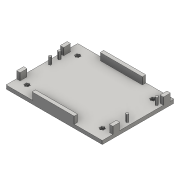
# Autodesk Inventor part: ROB-L-J-1
Saved by Autodesk Inventor 2016 (Build 200138000, 138)
## iProperties
Created: 2016-02-16
Part Number: ROB-L-J-1
Material: Generic
Document SubType Name: Modeling
Designer: admin
Density: 1 g/cm^3
Appearance: Default
Author: admin
Autodesk Inventor part; units mm, degrees
ref_plane "YZ Plane" through (0, 0, 0) normal (1, 0, 0) x (0, 1, 0)
ref_plane "XZ Plane" through (0, 0, 0) normal (0, 1, 0) x (-1, 0, 0)
ref_plane "XY Plane" through (0, 0, 0) normal (0, 0, 1) x (1, 0, 0)
sketch "Sketch1" plane through (0, 0, 0) normal (0, 0, 1) x (1, 0, 0)
  spline S0 degree 3 poles (79.3177, 119.4841) (79.3177, 118.5944) (78.5966, 117.873) (77.7073, 117.873) knots 0 0 0 0 1 1 1 1
  line L0 (79.3177, 119.4841) -> (79.3177, 118.5944) construction
  line L1 (79.3177, 118.5944) -> (78.5966, 117.873) construction
  line L2 (78.5966, 117.873) -> (77.7073, 117.873) construction
  spline S1 degree 3 poles (77.7073, 117.873) (76.818, 117.873) (76.0984, 118.5944) (76.0984, 119.4841) knots 0 0 0 0 1 1 1 1
  line L3 (77.7073, 117.873) -> (76.818, 117.873) construction
  line L4 (76.818, 117.873) -> (76.0984, 118.5944) construction
  line L5 (76.0984, 118.5944) -> (76.0984, 119.4841) construction
  spline S2 degree 3 poles (76.0984, 119.4841) (76.0984, 120.3739) (76.818, 121.0939) (77.7073, 121.0939) knots 0 0 0 0 1 1 1 1
  line L6 (76.0984, 119.4841) -> (76.0984, 120.3739) construction
  line L7 (76.0984, 120.3739) -> (76.818, 121.0939) construction
  line L8 (76.818, 121.0939) -> (77.7073, 121.0939) construction
  spline S3 degree 3 poles (77.7073, 121.0939) (78.5966, 121.0939) (79.3177, 120.3739) (79.3177, 119.4841) knots 0 0 0 0 1 1 1 1
  line L9 (77.7073, 121.0939) -> (78.5966, 121.0939) construction
  line L10 (78.5966, 121.0939) -> (79.3177, 120.3739) construction
  line L11 (79.3177, 120.3739) -> (79.3177, 119.4841) construction
  spline S4 degree 3 poles (79.3177, 47.5175) (79.3177, 46.6278) (78.5966, 45.9063) (77.7073, 45.9063) knots 0 0 0 0 1 1 1 1
  line L12 (79.3177, 47.5175) -> (79.3177, 46.6278) construction
  line L13 (79.3177, 46.6278) -> (78.5966, 45.9063) construction
  line L14 (78.5966, 45.9063) -> (77.7073, 45.9063) construction
  spline S5 degree 3 poles (77.7073, 45.9063) (76.818, 45.9063) (76.0984, 46.6278) (76.0984, 47.5175) knots 0 0 0 0 1 1 1 1
  line L15 (77.7073, 45.9063) -> (76.818, 45.9063) construction
  line L16 (76.818, 45.9063) -> (76.0984, 46.6278) construction
  line L17 (76.0984, 46.6278) -> (76.0984, 47.5175) construction
  spline S6 degree 3 poles (76.0984, 47.5175) (76.0984, 48.4072) (76.818, 49.1273) (77.7073, 49.1273) knots 0 0 0 0 1 1 1 1
  line L18 (76.0984, 47.5175) -> (76.0984, 48.4072) construction
  line L19 (76.0984, 48.4072) -> (76.818, 49.1273) construction
  line L20 (76.818, 49.1273) -> (77.7073, 49.1273) construction
  spline S7 degree 3 poles (77.7073, 49.1273) (78.5966, 49.1273) (79.3177, 48.4072) (79.3177, 47.5175) knots 0 0 0 0 1 1 1 1
  line L21 (77.7073, 49.1273) -> (78.5966, 49.1273) construction
  line L22 (78.5966, 49.1273) -> (79.3177, 48.4072) construction
  line L23 (79.3177, 48.4072) -> (79.3177, 47.5175) construction
  spline S8 degree 3 poles (186.2507, 47.5175) (186.2507, 46.6278) (185.531, 45.9063) (184.6417, 45.9063) knots 0 0 0 0 1 1 1 1
  line L24 (186.2507, 47.5175) -> (186.2507, 46.6278) construction
  line L25 (186.2507, 46.6278) -> (185.531, 45.9063) construction
  line L26 (185.531, 45.9063) -> (184.6417, 45.9063) construction
  spline S9 degree 3 poles (184.6417, 45.9063) (183.7524, 45.9063) (183.0327, 46.6278) (183.0327, 47.5175) knots 0 0 0 0 1 1 1 1
  line L27 (184.6417, 45.9063) -> (183.7524, 45.9063) construction
  line L28 (183.7524, 45.9063) -> (183.0327, 46.6278) construction
  line L29 (183.0327, 46.6278) -> (183.0327, 47.5175) construction
  spline S10 degree 3 poles (183.0327, 47.5175) (183.0327, 48.4072) (183.7524, 49.1273) (184.6417, 49.1273) knots 0 0 0 0 1 1 1 1
  line L30 (183.0327, 47.5175) -> (183.0327, 48.4072) construction
  line L31 (183.0327, 48.4072) -> (183.7524, 49.1273) construction
  line L32 (183.7524, 49.1273) -> (184.6417, 49.1273) construction
  spline S11 degree 3 poles (184.6417, 49.1273) (185.531, 49.1273) (186.2507, 48.4072) (186.2507, 47.5175) knots 0 0 0 0 1 1 1 1
  line L33 (184.6417, 49.1273) -> (185.531, 49.1273) construction
  line L34 (185.531, 49.1273) -> (186.2507, 48.4072) construction
  line L35 (186.2507, 48.4072) -> (186.2507, 47.5175) construction
  spline S12 degree 3 poles (186.2507, 119.4841) (186.2507, 118.5944) (185.531, 117.873) (184.6417, 117.873) knots 0 0 0 0 1 1 1 1
  line L36 (186.2507, 119.4841) -> (186.2507, 118.5944) construction
  line L37 (186.2507, 118.5944) -> (185.531, 117.873) construction
  line L38 (185.531, 117.873) -> (184.6417, 117.873) construction
  spline S13 degree 3 poles (184.6417, 117.873) (183.7524, 117.873) (183.0327, 118.5944) (183.0327, 119.4841) knots 0 0 0 0 1 1 1 1
  line L39 (184.6417, 117.873) -> (183.7524, 117.873) construction
  line L40 (183.7524, 117.873) -> (183.0327, 118.5944) construction
  line L41 (183.0327, 118.5944) -> (183.0327, 119.4841) construction
  spline S14 degree 3 poles (183.0327, 119.4841) (183.0327, 120.3739) (183.7524, 121.0939) (184.6417, 121.0939) knots 0 0 0 0 1 1 1 1
  line L42 (183.0327, 119.4841) -> (183.0327, 120.3739) construction
  line L43 (183.0327, 120.3739) -> (183.7524, 121.0939) construction
  line L44 (183.7524, 121.0939) -> (184.6417, 121.0939) construction
  spline S15 degree 3 poles (184.6417, 121.0939) (185.531, 121.0939) (186.2507, 120.3739) (186.2507, 119.4841) knots 0 0 0 0 1 1 1 1
  line L45 (184.6417, 121.0939) -> (185.531, 121.0939) construction
  line L46 (185.531, 121.0939) -> (186.2507, 120.3739) construction
  line L47 (186.2507, 120.3739) -> (186.2507, 119.4841) construction
  line L48 (73.2, 102) -> (67.7, 104.5)
  line L49 (67.7, 104.5) -> (67.7, 123.5)
  spline S16 degree 3 poles (67.7, 123.5) (67.7, 126.5) (70.7, 129.5) (73.7, 129.5) knots 0 0 0 0 1 1 1 1
  line L50 (67.7, 123.5) -> (67.7, 126.5) construction
  line L51 (67.7, 126.5) -> (70.7, 129.5) construction
  line L52 (70.7, 129.5) -> (73.7, 129.5) construction
  line L53 (73.7, 129.5) -> (188.7, 129.5)
  spline S17 degree 3 poles (188.7, 129.5) (191.7, 129.5) (194.7, 126.5) (194.7, 123.5) knots 0 0 0 0 1 1 1 1
  line L54 (188.7, 129.5) -> (191.7, 129.5) construction
  line L55 (191.7, 129.5) -> (194.7, 126.5) construction
  line L56 (194.7, 126.5) -> (194.7, 123.5) construction
  line L57 (194.7, 123.5) -> (194.7, 117.5)
  line L58 (194.7, 117.5) -> (189.2, 114)
  line L59 (189.2, 75) -> (194.7, 71.5)
  line L60 (194.7, 71.5) -> (194.7, 43.5)
  spline S18 degree 3 poles (194.7, 43.5) (194.7, 40.5) (191.7, 37.5) (188.7, 37.5) knots 0 0 0 0 1 1 1 1
  line L61 (194.7, 43.5) -> (194.7, 40.5) construction
  line L62 (194.7, 40.5) -> (191.7, 37.5) construction
  line L63 (191.7, 37.5) -> (188.7, 37.5) construction
  line L64 (188.7, 37.5) -> (73.7, 37.5)
  spline S19 degree 3 poles (73.7, 37.5) (70.7, 37.5) (67.7, 40.5) (67.7, 43.5) knots 0 0 0 0 1 1 1 1
  line L65 (73.7, 37.5) -> (70.7, 37.5) construction
  line L66 (70.7, 37.5) -> (67.7, 40.5) construction
  line L67 (67.7, 40.5) -> (67.7, 43.5) construction
  line L68 (67.7, 43.5) -> (67.7, 87.5)
  line L69 (67.7, 87.5) -> (73.2, 90)
  line L70 (73.7, 102) -> (73.7014, 90)
  line L71 (73.7014, 90) -> (73.2, 90)
  line L72 (189.2, 114) -> (188.7, 114)
  line L73 (188.7, 114) -> (188.7, 75)
  line L74 (188.7, 75) -> (189.2, 75)
  line L75 (73.2, 102) -> (73.7, 102)
  line L76 (62.7, 114.5) -> (62.7, 102)
  line L77 (62.7, 77.5) -> (62.7, 90)
  line L78 (199.7, 61.5) -> (199.7, 75)
  line L79 (199.7, 127.5) -> (199.7, 114)
  line L80 (99.7, 129.5) -> (159.7, 129.5)
  line L81 (159.7, 129.5) -> (159.7, 134.5)
  line L82 (159.7, 134.5) -> (99.7, 134.5)
  line L83 (99.7, 134.5) -> (99.7, 129.5)
  line L84 (99.7, 37.5) -> (159.7, 37.5)
  line L85 (159.7, 37.5) -> (159.7, 32.5)
  line L86 (159.7, 32.5) -> (99.7, 32.5)
  line L87 (99.7, 32.5) -> (99.7, 37.5)
  line L88 (62.7, 134.5) -> (199.7, 134.5)
  line L89 (199.7, 134.5) -> (199.7, 32.5)
  line L90 (199.7, 32.5) -> (62.7, 32.5)
  line L91 (62.7, 32.5) -> (62.7, 134.5)
  line L92 (67.7, 104.5) -> (66.4586, 101.7689)
  line L93 (66.4586, 101.7689) -> (69.1897, 100.5275)
  line L94 (69.1897, 100.5275) -> (70.4311, 103.2586)
  line L95 (70.4311, 103.2586) -> (67.7, 104.5)
  line L96 (67.7, 87.5) -> (70.4311, 88.7414)
  line L97 (70.4311, 88.7414) -> (69.1897, 91.4725)
  line L98 (69.1897, 91.4725) -> (66.4586, 90.2311)
  line L99 (66.4586, 90.2311) -> (67.7, 87.5)
  line L100 (194.7, 117.5) -> (192.169, 115.8894)
  line L101 (192.169, 115.8894) -> (193.7796, 113.3584)
  line L102 (193.7796, 113.3584) -> (196.3106, 114.969)
  line L103 (196.3106, 114.969) -> (194.7, 117.5)
  line L104 (194.7, 71.5) -> (192.169, 73.1106)
  line L105 (192.169, 73.1106) -> (193.7796, 75.6416)
  line L106 (193.7796, 75.6416) -> (196.3106, 74.031)
  line L107 (196.3106, 74.031) -> (194.7, 71.5)
  line L108 (67.7, 119.4841) -> (62.7, 119.4841)
  line L109 (62.7, 119.4841) -> (62.7, 109.4841)
  line L110 (62.7, 109.4841) -> (67.7, 109.4841)
  line L111 (67.7, 109.4841) -> (67.7, 119.4841)
  line L112 (67.7, 47.5175) -> (62.7, 47.5175)
  line L113 (62.7, 47.5175) -> (62.7, 57.5175)
  line L114 (62.7, 57.5175) -> (67.7, 57.5175)
  line L115 (67.7, 57.5175) -> (67.7, 47.5175)
  line L116 (194.7, 47.5175) -> (199.7, 47.5175)
  line L117 (199.7, 47.5175) -> (199.7, 57.5175)
  line L118 (199.7, 57.5175) -> (194.7, 57.5175)
  line L119 (194.7, 57.5175) -> (194.7, 47.5175)
  line L120 (194.7, 119.4841) -> (199.7, 119.4841)
  line L121 (199.7, 119.4841) -> (199.7, 129.5)
  line L122 (199.7, 129.5) -> (194.7, 129.5)
  line L123 (194.7, 129.5) -> (194.7, 119.4841)
  line L124 (184.6417, 47.5175) -> (181.7917, 47.5175)
  line L125 (181.7917, 49.1629) -> (184.6417, 50.8084)
  line L126 (184.6417, 50.8084) -> (187.4917, 49.1629)
  line L127 (187.4917, 49.1629) -> (187.4917, 45.872)
  line L128 (187.4917, 45.872) -> (184.6417, 44.2266)
  line L129 (184.6417, 44.2266) -> (181.7917, 45.872)
  line L130 (181.7917, 45.872) -> (181.7917, 49.1629)
  line L131 (182.0417, 49.5959) -> (187.7417, 46.305)
  line L132 (187.7417, 46.305) -> (187.2417, 45.439)
  line L133 (187.2417, 45.439) -> (181.5417, 48.7299)
  line L134 (181.5417, 48.7299) -> (182.0417, 49.5959)
  line L135 (182.0417, 49.5959) -> (187.2417, 45.439) construction
  line L136 (187.7417, 46.305) -> (181.5417, 48.7299) construction
  line L137 (186.9917, 45.5834) -> (187.4917, 46.4494)
  line L138 (187.4917, 45.872) -> (184.6417, 47.5175)
  circle A0 centre (187.2417, 46.0164) radius 0.5
  circle A1 centre (187.2417, 49.0186) radius 0.5
  circle A2 centre (184.6417, 50.5197) radius 0.5
  circle A3 centre (182.0417, 49.0186) radius 0.5
  circle A4 centre (182.0417, 46.0164) radius 0.5
  circle A5 centre (184.6417, 44.5153) radius 0.5
  circle A6 centre (184.6417, 47.5175) radius 2.5
  point P0 (0, 0)
  point P1 (77.7073, 121.0939)
  point P2 (79.3177, 119.4841)
  point P3 (77.7073, 119.4841)
  point P4 (184.6417, 119.4841)
  point P5 (77.7073, 49.1273)
  point P6 (79.3177, 47.5175)
  point P7 (77.7073, 47.5175)
  point P8 (77.7073, 119.4841)
  point P9 (186.9917, 49.4516)
  point P10 (184.1417, 50.5197)
  point P11 (181.7917, 48.5856)
  point P12 (182.2917, 45.5834)
  point P13 (185.1417, 44.5153)
  dimension "d9" = 60
  dimension "d10" = 5
  dimension "d11" = 5
  dimension "d44" = 3
  dimension "d45" = 3
  dimension "d46" = 3
  dimension "d47" = 3
  dimension "d48" = 3
  dimension "d49" = 3
  dimension "d50" = 3
  dimension "d51" = 3
  dimension "d52" = 10
  dimension "d53" = 10
  dimension "d56" = 10
  dimension "d62" = 5
  dimension "d63" = 2.85
  dimension "d64" = 1
  dimension "d67" = 360
  dimension "d71" = 5
  constraints: 158 end point, 24 parallel, 22 point on line, 13 perpendicular, 12 coincident, 8 horizontal, 4 midpoint, 2 horizontal alignment, 1 centre point, 108 other
  measures "d9" distance of L82.end L81.end
  measures "d10" distance of L81.end L80.end
  measures "d11" distance of L84.end L85.end
  measures "d44" distance of L49.start L92.end
  measures "d45" distance of L93.end L92.end
  measures "d46" distance of L69.start L96.end
  measures "d47" distance of L97.end L96.end
  measures "d48" distance of L58.start L100.end
  measures "d49" distance of L101.end L100.end
  measures "d50" distance of L60.start L104.end
  measures "d51" distance of L104.end L105.end
  measures "d52" distance of L109.end L108.end
  measures "d53" distance of L112.end L113.end
  measures "d56" distance of L117.end L116.end
  measures "d62" distance between parallel lines of L78 L60
  measures "d63" distance of L124.start L124.end
  measures "d64" distance of L131.end L132.end
  measures "d71" diameter of A6
sketch "HOLES1" plane through (0, 0, 0) normal (0, 0, 1) x (1, 0, 0)
  spline S0 degree 3 poles (78.0941, 113.5873) (78.0941, 112.8755) (77.5173, 112.2984) (76.8059, 112.2984) knots 0 0 0 0 1 1 1 1
  line L0 (78.0941, 113.5873) -> (78.0941, 112.8755) construction
  line L1 (78.0941, 112.8755) -> (77.5173, 112.2984) construction
  line L2 (77.5173, 112.2984) -> (76.8059, 112.2984) construction
  spline S1 degree 3 poles (76.8059, 112.2984) (76.0944, 112.2984) (75.5187, 112.8755) (75.5187, 113.5873) knots 0 0 0 0 1 1 1 1
  line L3 (76.8059, 112.2984) -> (76.0944, 112.2984) construction
  line L4 (76.0944, 112.2984) -> (75.5187, 112.8755) construction
  line L5 (75.5187, 112.8755) -> (75.5187, 113.5873) construction
  spline S2 degree 3 poles (75.5187, 113.5873) (75.5187, 114.2991) (76.0944, 114.8751) (76.8059, 114.8751) knots 0 0 0 0 1 1 1 1
  line L6 (75.5187, 113.5873) -> (75.5187, 114.2991) construction
  line L7 (75.5187, 114.2991) -> (76.0944, 114.8751) construction
  line L8 (76.0944, 114.8751) -> (76.8059, 114.8751) construction
  spline S3 degree 3 poles (76.8059, 114.8751) (77.5173, 114.8751) (78.0941, 114.2991) (78.0941, 113.5873) knots 0 0 0 0 1 1 1 1
  line L9 (76.8059, 114.8751) -> (77.5173, 114.8751) construction
  line L10 (77.5173, 114.8751) -> (78.0941, 114.2991) construction
  line L11 (78.0941, 114.2991) -> (78.0941, 113.5873) construction
  spline S4 degree 3 poles (78.0941, 56.014) (78.0941, 55.3022) (77.5173, 54.7251) (76.8059, 54.7251) knots 0 0 0 0 1 1 1 1
  line L12 (78.0941, 56.014) -> (78.0941, 55.3022) construction
  line L13 (78.0941, 55.3022) -> (77.5173, 54.7251) construction
  line L14 (77.5173, 54.7251) -> (76.8059, 54.7251) construction
  spline S5 degree 3 poles (76.8059, 54.7251) (76.0944, 54.7251) (75.5187, 55.3022) (75.5187, 56.014) knots 0 0 0 0 1 1 1 1
  line L15 (76.8059, 54.7251) -> (76.0944, 54.7251) construction
  line L16 (76.0944, 54.7251) -> (75.5187, 55.3022) construction
  line L17 (75.5187, 55.3022) -> (75.5187, 56.014) construction
  spline S6 degree 3 poles (75.5187, 56.014) (75.5187, 56.7258) (76.0944, 57.3018) (76.8059, 57.3018) knots 0 0 0 0 1 1 1 1
  line L18 (75.5187, 56.014) -> (75.5187, 56.7258) construction
  line L19 (75.5187, 56.7258) -> (76.0944, 57.3018) construction
  line L20 (76.0944, 57.3018) -> (76.8059, 57.3018) construction
  spline S7 degree 3 poles (76.8059, 57.3018) (77.5173, 57.3018) (78.0941, 56.7258) (78.0941, 56.014) knots 0 0 0 0 1 1 1 1
  line L21 (76.8059, 57.3018) -> (77.5173, 57.3018) construction
  line L22 (77.5173, 57.3018) -> (78.0941, 56.7258) construction
  line L23 (78.0941, 56.7258) -> (78.0941, 56.014) construction
  spline S8 degree 3 poles (163.6406, 56.014) (163.6406, 55.3022) (163.0648, 54.7251) (162.3534, 54.7251) knots 0 0 0 0 1 1 1 1
  line L24 (163.6406, 56.014) -> (163.6406, 55.3022) construction
  line L25 (163.6406, 55.3022) -> (163.0648, 54.7251) construction
  line L26 (163.0648, 54.7251) -> (162.3534, 54.7251) construction
  spline S9 degree 3 poles (162.3534, 54.7251) (161.6419, 54.7251) (161.0662, 55.3022) (161.0662, 56.014) knots 0 0 0 0 1 1 1 1
  line L27 (162.3534, 54.7251) -> (161.6419, 54.7251) construction
  line L28 (161.6419, 54.7251) -> (161.0662, 55.3022) construction
  line L29 (161.0662, 55.3022) -> (161.0662, 56.014) construction
  spline S10 degree 3 poles (161.0662, 56.014) (161.0662, 56.7258) (161.6419, 57.3018) (162.3534, 57.3018) knots 0 0 0 0 1 1 1 1
  line L30 (161.0662, 56.014) -> (161.0662, 56.7258) construction
  line L31 (161.0662, 56.7258) -> (161.6419, 57.3018) construction
  line L32 (161.6419, 57.3018) -> (162.3534, 57.3018) construction
  spline S11 degree 3 poles (162.3534, 57.3018) (163.0648, 57.3018) (163.6406, 56.7258) (163.6406, 56.014) knots 0 0 0 0 1 1 1 1
  line L33 (162.3534, 57.3018) -> (163.0648, 57.3018) construction
  line L34 (163.0648, 57.3018) -> (163.6406, 56.7258) construction
  line L35 (163.6406, 56.7258) -> (163.6406, 56.014) construction
  spline S12 degree 3 poles (163.6406, 113.5873) (163.6406, 112.8755) (163.0648, 112.2984) (162.3534, 112.2984) knots 0 0 0 0 1 1 1 1
  line L36 (163.6406, 113.5873) -> (163.6406, 112.8755) construction
  line L37 (163.6406, 112.8755) -> (163.0648, 112.2984) construction
  line L38 (163.0648, 112.2984) -> (162.3534, 112.2984) construction
  spline S13 degree 3 poles (162.3534, 112.2984) (161.6419, 112.2984) (161.0662, 112.8755) (161.0662, 113.5873) knots 0 0 0 0 1 1 1 1
  line L39 (162.3534, 112.2984) -> (161.6419, 112.2984) construction
  line L40 (161.6419, 112.2984) -> (161.0662, 112.8755) construction
  line L41 (161.0662, 112.8755) -> (161.0662, 113.5873) construction
  spline S14 degree 3 poles (161.0662, 113.5873) (161.0662, 114.2991) (161.6419, 114.8751) (162.3534, 114.8751) knots 0 0 0 0 1 1 1 1
  line L42 (161.0662, 113.5873) -> (161.0662, 114.2991) construction
  line L43 (161.0662, 114.2991) -> (161.6419, 114.8751) construction
  line L44 (161.6419, 114.8751) -> (162.3534, 114.8751) construction
  spline S15 degree 3 poles (162.3534, 114.8751) (163.0648, 114.8751) (163.6406, 114.2991) (163.6406, 113.5873) knots 0 0 0 0 1 1 1 1
  line L45 (162.3534, 114.8751) -> (163.0648, 114.8751) construction
  line L46 (163.0648, 114.8751) -> (163.6406, 114.2991) construction
  line L47 (163.6406, 114.2991) -> (163.6406, 113.5873) construction
  constraints: 48 other
sketch "OUTLINE1" plane through (0, 0, 0) normal (0, 0, 1) x (1, 0, 0)
  line L0 (73.2, 99.6) -> (68.8, 101.6)
  line L1 (68.8, 101.6) -> (68.8, 116.8)
  spline S0 degree 3 poles (68.8, 116.8) (68.8, 119.2) (71.2, 121.6) (73.6, 121.6) knots 0 0 0 0 1 1 1 1
  line L2 (68.8, 116.8) -> (68.8, 119.2) construction
  line L3 (68.8, 119.2) -> (71.2, 121.6) construction
  line L4 (71.2, 121.6) -> (73.6, 121.6) construction
  line L5 (73.6, 121.6) -> (165.6, 121.6)
  spline S1 degree 3 poles (165.6, 121.6) (168, 121.6) (170.4, 119.2) (170.4, 116.8) knots 0 0 0 0 1 1 1 1
  line L6 (165.6, 121.6) -> (168, 121.6) construction
  line L7 (168, 121.6) -> (170.4, 119.2) construction
  line L8 (170.4, 119.2) -> (170.4, 116.8) construction
  line L9 (170.4, 116.8) -> (170.4, 112)
  line L10 (170.4, 112) -> (166, 109.2)
  line L11 (166, 78) -> (170.4, 75.2)
  line L12 (170.4, 75.2) -> (170.4, 52.8)
  spline S2 degree 3 poles (170.4, 52.8) (170.4, 50.4) (168, 48) (165.6, 48) knots 0 0 0 0 1 1 1 1
  line L13 (170.4, 52.8) -> (170.4, 50.4) construction
  line L14 (170.4, 50.4) -> (168, 48) construction
  line L15 (168, 48) -> (165.6, 48) construction
  line L16 (165.6, 48) -> (73.6, 48)
  spline S3 degree 3 poles (73.6, 48) (71.2, 48) (68.8, 50.4) (68.8, 52.8) knots 0 0 0 0 1 1 1 1
  line L17 (73.6, 48) -> (71.2, 48) construction
  line L18 (71.2, 48) -> (68.8, 50.4) construction
  line L19 (68.8, 50.4) -> (68.8, 52.8) construction
  line L20 (68.8, 52.8) -> (68.8, 88)
  line L21 (68.8, 88) -> (73.2, 90)
  constraints: 20 end point, 12 other
sketch "OUTLINE2" plane through (0, 0, 0) normal (0, 0, 1) x (1, 0, 0)
  line L0 (73.6, 99.6) -> (73.6011, 90)
  line L1 (73.6011, 90) -> (73.2, 90)
  line L2 (166, 109.2) -> (165.6, 109.2)
  line L3 (165.6, 109.2) -> (165.6, 78)
  line L4 (165.6, 78) -> (166, 78)
  line L5 (73.2, 99.6) -> (73.6, 99.6)
  constraints: 12 end point
extrude "Extrusion2" add sketch "Sketch1" against normal blind 5 contours S0 S1 S2 S3 | S4 S5 S6 S7 | S11 S10 L131 A6 S8 | S8 L131 S10 S11 | L131 A6 L138 S8 | S8 L138 L124 L133 S10 L131 | L138 A6 L133 S8 | S8 L133 L124 L138 | S10 L133 A6 L131 | A6 L131 L125 A2 L126 A1 L127 | L131 A0 A6 | L133 A6 L124 S9 S8 | S8 S9 L124 L133 | A0 L137 L138 | L138 L137 A0 | A0 L133 A6 | L133 L124 S10 | S10 L124 A6 L133 | A6 L133 A3 L131 | A0 L132 L127 | L127 L138 L137 | L131 L132 A0 | L133 L128 A5 L129 A4 L130 L124 A6 | L138 L128 L137 | A0 L132 L133 | L128 L132 A0 | A6 L124 L130 L133 | A3 L130 L125 | A3 L134 L131 | L125 L134 A3 | L132 A0 | A1 L126 L127 | L127 L126 A1 | A5 L129 L128 | L128 L129 A5 | A3 L134 L130 | L133 L134 A3 | L134 A3 | A2 L126 L125 | L125 L126 A2 | A4 L129 L130 | L130 L129 A4 | S12 S13 S14 S15 | L75 L70 L71 L69 L97 L98 L99 L68 L114 L91 L77 L76 L110 L49 L92 L93 L94 L48 | L48 L49 S16 L53 S17 L57 L58 L72 L73 L74 L59 L60 S18 L64 S19 L68 L69 L71 L70 L75 | L94 L93 L92 L48 | L110 L76 L91 L108 L49 | L108 L91 L88 L83 L53 S16 L49 | L69 L99 L98 L97 | L68 L112 L91 L114 | L83 L82 L81 L53 | L68 S19 L64 L87 L90 L91 L112 | L81 L88 L89 L122 L123 S17 L53 | L123 L122 L89 L79 L120 L57 | L64 L85 L86 L87 | L120 L79 L89 L78 L118 L60 L107 L106 L105 L59 L74 L73 L72 L58 L101 L102 L103 L57 | L64 S18 L60 L116 L89 L90 L85 | L103 L102 L101 L58 | L116 L60 L118 L89 | L59 L105 L106 L107
fillet "Fillet1" radius 0.5 4 edges at (199.7, 32.5, -2.5) (199.7, 134.5, -2.5) (62.7, 134.5, -2.5) (62.7, 32.5, -2.5)
extrude "Extrusion7" add sketch "Sketch1" along normal blind 10 contours L94 L93 L92 L48 | L110 L76 L91 L108 L49 | L69 L99 L98 L97 | L68 L112 L91 L114 | L83 L82 L81 L53 | L123 L122 L89 L79 L120 L57 | L64 L85 L86 L87 | L103 L102 L101 L58 | L116 L60 L118 L89 | L59 L105 L106 L107
fillet "Fillet3" radius 0.5 39 edges at (99.7, 129.5, 5) (159.7, 129.5, 5) (199.7, 119.4841, 5) (193.7796, 113.3584, 5) (196.3106, 114.969, 5) (192.169, 73.1106, 5) (194.7, 71.5, 5) (194.7, 47.5175, 5) (199.7, 47.5175, 5) (159.7, 32.5, 5) (99.7, 32.5, 5) (62.7, 47.5175, 5) (67.7, 47.5175, 5) (62.7, 109.4841, 5) (69.1897, 100.5275, 5) (67.7, 87.5, 5) (66.4586, 90.2311, 5) (66.4586, 101.7689, 5) (67.7, 109.4841, 5) (194.7, 119.4841, 5) (192.169, 115.8894, 5) (159.7, 37.5, 5) (199.7, 57.5175, 5) (196.3106, 74.031, 5) (193.7796, 75.6416, 5) (199.7, 129.5, 5) (194.7, 129.5, 5) (159.7, 134.5, 5) (99.7, 37.5, 5) (99.7, 134.5, 5) (62.7, 119.4841, 5) (67.7, 119.4841, 5) (67.7, 104.5, 5) (70.4311, 103.2586, 5) (69.1897, 91.4725, 5) (62.7, 57.5175, 5) (67.7, 57.5175, 5) (194.7, 57.5175, 5) (70.4311, 88.7414, 5)
extrude "Extrusion8" cut sketch "Sketch1" against normal blind 2.3 contours S11 S10 L131 A6 S8 | S8 L131 S10 S11 | L131 A6 L138 S8 | S8 L138 L124 L133 S10 L131 | L138 A6 L133 S8 | S8 L133 L124 L138 | S10 L133 A6 L131 | A6 L131 L125 A2 L126 A1 L127 | L131 A0 A6 | L133 A6 L124 S9 S8 | S8 S9 L124 L133 | A0 L137 L138 | L138 L137 A0 | A0 L133 A6 | L133 L124 S10 | S10 L124 A6 L133 | A6 L133 A3 L131 | A0 L132 L127 | L127 L138 L137 | L133 L128 A5 L129 A4 L130 L124 A6 | L138 L128 L137 | L128 L132 A0 | A6 L124 L130 L133 | A3 L130 L125 | L125 L134 A3 | L132 A0 | A1 L126 L127 | L127 L126 A1 | A5 L129 L128 | L128 L129 A5 | A3 L134 L130 | L134 A3 | A2 L126 L125 | L125 L126 A2 | A4 L129 L130 | L130 L129 A4
extrude "Extrusion9" cut sketch "Sketch1" against normal blind 10 contours S11 S10 L131 A6 S8 | S8 L131 S10 S11 | L131 A6 L138 S8 | S8 L138 L124 L133 S10 L131 | L138 A6 L133 S8 | S8 L133 L124 L138 | S10 L133 A6 L131 | L133 A6 L124 S9 S8 | S8 S9 L124 L133 | L133 L124 S10 | S10 L124 A6 L133
pattern_linear "Rectangular Pattern2" count 2 spacing 72 along (0.0000003, 1, 0) count 2 spacing 107 along (-1, 0, 0) of "Extrusion8", "Extrusion9"
body "Solid1"
